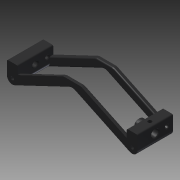
# Autodesk Inventor part: Front mount
Saved by Autodesk Inventor 2015 (Build 190159000, 159)
## iProperties
Created: 2016-10-31
Part Number: Front mount
Material: ABS Plastic
Document SubType Name: Modeling
Designer: James Yelland
Density: 1.06 g/cm^3
Appearance: Smooth - White
Mass: 7.98828 g
Surface Area: 62.2612 cm^2
Volume: 7.53611 cm^3
Author: James Yelland
Autodesk Inventor part; units mm, degrees
ref_plane "YZ Plane" through (0, 0, 0) normal (1, 0, 0) x (0, 1, 0)
ref_plane "XZ Plane" through (0, 0, 0) normal (0, 1, 0) x (-1, 0, 0)
sketch "Sketch2" plane through (0, 0, 0) normal (0, 1, 0) x (-1, 0, 0)
  circle A0 centre (50.479367, -84.432507) radius 1.4
  circle A1 centre (-50.479367, -84.432507) radius 1.4
  arc A2 (0, -65.970621) -> (-2.364635, -66.504889) centre (0, -71.470621) ccw
  arc A3 (2.364635, -66.504889) -> (0, -65.970621) centre (0, -71.470621) ccw
  line L0 (2.364635, -66.504889) -> (48.544666, -88.495379)
  line L1 (-2.364635, -66.504889) -> (-48.544666, -88.495379)
  arc A4 (48.544666, -88.495379) -> (47.928167, -80.725571) centre (50.479367, -84.432507) ccw
  arc A5 (-47.928167, -80.725571) -> (-48.544666, -88.495379) centre (-50.479367, -84.432507) ccw
  line L2 (-8.449668, -61.926286) -> (-47.928167, -80.725571)
  line L3 (8.449668, -61.926286) -> (47.928167, -80.725571)
  line L4 (-6.3, -61.440588) -> (6.3, -61.440588)
  arc A6 (-6.3, -61.440588) -> (-8.449668, -61.926286) centre (-6.3, -66.440588) ccw
  arc A7 (8.449668, -61.926286) -> (6.3, -61.440588) centre (6.3, -66.440588) ccw
  point P0 (0, 0)
  point P1 (52.5, -90.932667)
  dimension "d14" = 2.8
  dimension "d15" = 2.8
  dimension "d20" = 6.75
  dimension "d21" = 6.75
  dimension "d22" = 5
  constraints: 12 point on circle, 10 end point, 8 centre point, 4 tangent, 3 coincident, 1 equal radius, 1 horizontal
  measures "d14" diameter of A0
  measures "d15" diameter of A1
  measures "d20" distance between parallel lines of L1 L2
  measures "d21" distance between parallel lines of L3 L0
  measures "d22" radius of A6
extrude "Extrusion1" add sketch "Sketch2" along normal blind 3
sketch "Sketch3" plane through (0, 3, 0) normal (0, 1, 0) x (1, 0, 0)
  circle A0 centre (50.479367, 84.432507) radius 1.4
  circle A1 centre (-50.479367, 84.432507) radius 1.4
  line L0 (-2.364635, 66.504889) -> (-48.544666, 88.495379)
  arc A2 (-48.544666, 88.495379) -> (-47.928167, 80.725571) centre (-50.479367, 84.432507) ccw
  arc A3 (47.928167, 80.725571) -> (48.544666, 88.495379) centre (50.479367, 84.432507) ccw
  line L1 (48.544666, 88.495379) -> (2.364635, 66.504889)
  arc A4 (-2.364635, 66.504889) -> (2.364635, 66.504889) centre (0, 71.470621) ccw
  circle A5 centre (-50.479367, 84.432507) radius 1.4
  circle A6 centre (-50.479367, 84.432507) radius 4.5
  circle A7 centre (50.479367, 84.432507) radius 1.4
  circle A8 centre (50.479367, 84.432507) radius 4.5
  line L2 (-47.928167, 80.725571) -> (-8.449668, 61.926286)
  arc A9 (-8.449668, 61.926286) -> (-6.3, 61.440588) centre (-6.3, 66.440588) ccw
  line L3 (-6.3, 61.440588) -> (6.3, 61.440588)
  arc A10 (6.3, 61.440588) -> (8.449668, 61.926286) centre (6.3, 66.440588) ccw
  line L4 (8.449668, 61.926286) -> (47.928167, 80.725571)
  point P0 (0, 0)
  constraints: 4 centre point, 4 coincident, 4 concentric
extrude "Extrusion2" add sketch "Sketch3" along normal blind 24 contours A6 A2 | A3 A8
sketch "Sketch4" plane through (-50.479367, 27, -84.432507) normal (0, 1, 0) x (1, 0, 0)
  arc A0 (2.5512, -3.706936) -> (1.934701, 4.062872) centre (0, 0) ccw
  arc A1 (99.024032, 4.062872) -> (98.407533, -3.706936) centre (100.958733, 0) ccw
  line L0 (99.024032, 4.062872) -> (52.844001, -17.927619)
  arc A2 (48.114732, -17.927619) -> (52.844001, -17.927619) centre (50.479367, -12.961886) ccw
  line L1 (48.114732, -17.927619) -> (1.934701, 4.062872)
  circle A3 centre (0, 0) radius 4.5
  circle A4 centre (100.958733, 0) radius 1.4
  circle A5 centre (100.958733, 0) radius 4.5
  circle A6 centre (0, 0) radius 1.4
  line L2 (2.5512, -3.706936) -> (42.029699, -22.506222)
  arc A7 (42.029699, -22.506222) -> (44.179367, -22.991919) centre (44.179367, -17.991919) ccw
  line L3 (44.179367, -22.991919) -> (56.779367, -22.991919)
  arc A8 (56.779367, -22.991919) -> (58.929035, -22.506222) centre (56.779367, -17.991919) ccw
  line L4 (58.929035, -22.506222) -> (98.407533, -3.706936)
  point P0 (50.479367, -84.432507)
extrude "Extrusion3" add sketch "Sketch4" along normal blind 3
fillet "Fillet1" radius 1 17 edges at (-1.2121, 3, -66.1059) (1.2121, 3, -66.1059) (-25.4547, 3, -77.5001) (25.4547, 3, -77.5001) (0, 27, -65.9706) (25.4547, 27, -77.5001) (-25.4547, 27, -77.5001) (7.4019, 3, -61.5635) (28.1889, 3, -71.3259) (-7.4019, 3, -61.5635) (-28.1889, 3, -71.3259) (0, 3, -61.4406) (7.4019, 27, -61.5635) (28.1889, 27, -71.3259) (-7.4019, 27, -61.5635) (-28.1889, 27, -71.3259) (0, 27, -61.4406)
ref_plane "Work Plane1" through (50.479367, 0, -79.932507) normal (0, 0, 1) x (1, 0, 0)
sketch "Sketch5" plane through (50.479367, 0, -79.932507) normal (0, 0, 1) x (1, 0, 0)
  line L0 (4.5, 0) -> (4.5, 30)
  line L1 (-4.5, 3) -> (-4.5, 27)
  line L2 (4.5, 30) -> (-4.5, 30)
  line L3 (-4.5, 30) -> (-4.5, 0)
  line L4 (-4.5, 0) -> (4.5, 0)
  line L5 (4.5, 0) -> (4.5, 30)
  line L6 (-105.458733, 0) -> (-105.458733, 30)
  line L7 (-98.407533, 30) -> (-105.458733, 30)
  line L8 (-105.458733, 30) -> (-96.458733, 30)
  line L9 (-96.458733, 30) -> (-96.458733, 0)
  line L10 (-96.458733, 0) -> (-105.458733, 0)
  line L11 (-105.458733, 0) -> (-105.458733, 30)
  point P0 (-50.479367, 0)
  point P1 (-99.024032, 30)
  dimension "d23" = 30
  dimension "d24" = 9
  dimension "d25" = 30
  constraints: 16 end point, 4 parallel, 2 horizontal, 2 perpendicular, 1 point on line
  measures "d23" distance of L3.end L2.end
  measures "d24" distance of L9.end L10.end
  measures "d25" distance of L8.end L9.end
extrude "Extrusion4" add sketch "Sketch5" along normal blind 7 and the other way blind 4.5
sketch "Sketch6" plane through (-50.479367, 30, -84.432507) normal (0, 1, 0) x (1, 0, 0)
  line L0 (1.4, 0) -> (-1.4, 0)
  circle A0 centre (0, 0) radius 1.4
  line L1 (102.358733, 0) -> (99.558733, 0)
  circle A1 centre (100.958733, 0) radius 1.4
  point P0 (50.479367, -84.432507)
  constraints: 2 centre point, 2 midpoint
extrude "Extrusion5" cut sketch "Sketch6" against normal through all
fillet "Fillet2" radius 1 4 edges at (54.9794, 15, -72.9325) (45.9794, 15, -72.9325) (-45.9794, 15, -72.9325) (-54.9794, 15, -72.9325)
sketch "Sketch7" plane through (54.979367, 0, -84.432507) normal (1, 0, 0) x (0, 0, -1)
  line L0 (-11.5, 30) -> (-11.5, 15)
  line L1 (-11.5, 30) -> (-11.5, 0) projected
  line L2 (-11.5, 15) -> (-5, 15)
  circle A0 centre (-5, 15) radius 3.1
  point P0 (-84.432507, 0)
  dimension "d33" = 15
  dimension "d34" = 6.5
  dimension "d35" = 6.2
  constraints: 4 end point, 1 centre point, 1 coincident, 1 midpoint, 1 perpendicular
  measures "d33" distance of L0.start L0.end
  measures "d34" distance of L0.end L2.end
  measures "d35" diameter of A0
extrude "Extrusion6" cut sketch "Sketch7" against normal blind 10
sketch "Sketch8" plane through (45.979367, 3, -84.432507) normal (-1, 0, 0) x (0, 0, 1)
  circle A0 centre (5, 12) radius 3.1 projected
  circle A1 centre (5, 12) radius 3.1
  circle A2 centre (5, 12) radius 4.5
  point P0 (84.432507, -3)
  dimension "d39" = 9
  constraints: 2 centre point, 2 coincident, 1 concentric
  measures "d39" diameter of A2
extrude "Extrusion7" add sketch "Sketch8" along normal blind 5
chamfer "Chamfer1" distance 0.75 angle 45 1 edges at (40.9794, 15, -83.9325)
sketch "Sketch9" plane through (50.479367, 0, -72.932507) normal (0, 0, 1) x (1, 0, 0)
  line L0 (-3.5, 0) -> (-3.5, 30) projected
  line L1 (-3.5, 0) -> (3.5, 0) projected
  line L2 (3.5, 30) -> (3.5, 0) projected
  line L3 (3.5, 30) -> (-3.5, 30) projected
  line L4 (0, 30) -> (0, 15)
  circle A0 centre (0, 15) radius 1.5
  point P0 (-50.479367, 0)
  dimension "d45" = 15
  dimension "d46" = 3
  constraints: 2 end point, 1 centre point, 1 coincident, 1 midpoint, 1 vertical
  measures "d45" distance of L4.start L4.end
  measures "d46" diameter of A0
extrude "Extrusion8" cut sketch "Sketch9" against normal up to next contours A0
sketch "Sketch10" plane through (54.979367, 0, -84.432507) normal (1, 0, 0) x (0, 0, -1)
  circle A0 centre (-5, 15) radius 3.1 projected
  line L0 (-10.5, 0) -> (-10.5, 30) projected
  line L1 (0, 0) -> (-10.5, 0) projected
  line L2 (0, 30) -> (0, 0) projected
  line L3 (-10.5, 30) -> (0, 30) projected
  line L4 (-5, 15) -> (-5, 25)
  circle A1 centre (-5, 25) radius 1.5
  point P0 (-84.432507, 0)
  dimension "d49" = 10
  dimension "d50" = 3
  constraints: 2 end point, 1 centre point, 1 coincident, 1 vertical
  measures "d49" distance of L4.start L4.end
  measures "d50" diameter of A1
extrude "Extrusion9" cut sketch "Sketch10" against normal blind 10 contours A1
sketch "Sketch11" plane through (-45.979367, 3, -84.432507) normal (1, 0, 0) x (0, 0, -1)
  circle A0 centre (-5, 12) radius 3.1 projected
  circle A1 centre (-5, 12) radius 2.25
  point P0 (-84.432507, -3)
  dimension "d53" = 4.5
  constraints: 1 centre point, 1 coincident
  measures "d53" diameter of A1
extrude "Extrusion10" cut sketch "Sketch11" against normal blind 5 contours A1
chamfer "Chamfer2" distance 0.5 angle 45 1 edges at (-45.9794, 15, -77.1825)
sketch "Sketch12" plane through (-50.979367, 15, -79.432507) normal (1, 0, 0) x (0, 0, -1)
  circle A0 centre (0, 0) radius 2.25 projected
  circle A1 centre (0, 0) radius 2.25 projected
  line L0 (0, 0) -> (0, 1.25)
  line L1 (0, 0) -> (0, -1.25)
  circle A2 centre (0, 1.25) radius 0.4
  circle A3 centre (0, -1.25) radius 0.4
  point P0 (-79.432507, -15)
  dimension "d59" = 1.25
  dimension "d60" = 1.25
  dimension "d61" = 0.8
  dimension "d62" = 0.8
  constraints: 4 end point, 2 centre point, 2 coincident, 2 vertical
  measures "d59" distance of L0.start L0.end
  measures "d60" distance of L0.start L1.end
  measures "d61" diameter of A2
  measures "d62" diameter of A3
extrude "Extrusion11" cut sketch "Sketch12" against normal through all contours A2 | A3
sketch "Sketch13" plane through (-45.979367, 3, -84.432507) normal (1, 0, 0) x (0, 0, -1)
  circle A0 centre (-5, 22) radius 1.5 projected
  point P0 (-84.432507, -3)
extrude "Extrusion12" cut sketch "Sketch13" against normal through all
chamfer "Chamfer3" distance 0.5 angle 45 5 edges at (54.9794, 15, -76.3325) (54.9794, 25, -77.9325) (-45.9794, 25, -77.9325) (-54.9794, 25, -77.9325) (45.9794, 25, -77.9325)
body "Solid1"
